# Autodesk Inventor part: STAND-OFF
Saved by Autodesk Inventor 2016 SP1 (Build 200210100, 210)
## iProperties
Created: 2015-11-19
Part Number: STAND-OFF
Material: Generic
Document SubType Name: Modeling
Designer: PhillipD
Density: 1 g/cm^3
Appearance: STAND-OFF, STAND-OFF
Author: PhillipD
Autodesk Inventor part; units mm, degrees
ref_plane "YZ Plane" through (0, 0, 0) normal (1, 0, 0) x (0, 1, 0)
ref_plane "XZ Plane" through (0, 0, 0) normal (0, 1, 0) x (-1, 0, 0)
ref_plane "XY Plane" through (0, 0, 0) normal (0, 0, 1) x (1, 0, 0)
sketch "STAND-OFF, STAND-OFF_56" plane through (0, 0, 0) normal (0, 0, 1) x (1, 0, 0)
  line L0 (-2.8575, 2.8575) -> (2.8575, 2.8575)
  line L1 (2.8575, 2.8575) -> (2.8575, -2.8575)
  line L2 (2.8575, -2.8575) -> (-2.8575, -2.8575)
  line L3 (-2.8575, -2.8575) -> (-2.8575, 2.8575)
  constraints: 8 end point
extrude "Extrusion1" add sketch "STAND-OFF, STAND-OFF_56" along normal blind 1
body "Solid1"
